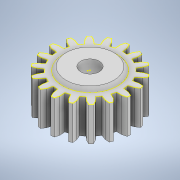
# Autodesk Inventor part: metal_gearbox_gear
Saved by Autodesk Inventor 2020 (Build 240168000, 168)
## iProperties
Created: 2020-01-28
Part Number: metal_gearbox_gear
Material: Generic
Document SubType Name: Modeling
Designer: erwin
Density: 1 g/cm^3
Appearance: Default
Author: erwin
Autodesk Inventor part; units mm, degrees
ref_plane "YZ Plane" through (0, 0, 0) normal (1, 0, 0) x (0, 1, 0)
ref_plane "XZ Plane" through (0, 0, 0) normal (0, 1, 0) x (-1, 0, 0)
ref_plane "XY Plane" through (0, 0, 0) normal (0, 0, 1) x (1, 0, 0)
sketch "Sketch1" plane through (0, 0, 0) normal (0, 1, 0) x (-1, 0, 0)
  line L0 (-38.3271, 50.3843) -> (32.9901, 50.3843) construction
  line L1 (32.9901, 50.3843) -> (32.9901, -44.7054) construction
  line L2 (32.9901, -44.7054) -> (-38.3271, -44.7054) construction
  line L3 (-38.3271, -44.7054) -> (-38.3271, 50.3843) construction
  circle A0 centre (-0.1536, -0.2457) radius 1.55
  arc A1 (6.806, -0.9968) -> (6.8429, -0.4678) centre (-0.1536, -0.2457) ccw
  circle A2 centre (-0.1536, -0.2457) radius 3.9907
  circle A3 centre (-0.1536, -0.2457) radius 4.6909
  circle A4 centre (-0.1536, -0.2457) radius 5.4294
  line L4 (5.1931, -1.1899) -> (6.0958, -1.1899)
  line L5 (6.0958, -1.1899) -> (6.806, -0.9968)
  line L6 (6.8429, -0.4678) -> (6.1696, -0.1708)
  line L7 (5.2729, -0.0666) -> (6.1696, -0.1708)
  line L8 (5.1936, 0.6958) -> (6.0419, 1.0045)
  line L9 (4.8844, 1.7785) -> (5.7626, 1.9874)
  line L10 (6.4969, 1.9385) -> (5.7626, 1.9874)
  arc A5 (6.6432, 1.4288) -> (6.4969, 1.9385) centre (-0.1536, -0.2457) ccw
  line L11 (6.0419, 1.0045) -> (6.6432, 1.4288)
  line L12 (4.5491, 2.4678) -> (5.2407, 3.0481)
  line L13 (3.8882, 3.3796) -> (4.6421, 3.8762)
  line L14 (5.3488, 4.0814) -> (4.6421, 3.8762)
  arc A6 (5.6606, 3.6524) -> (5.3488, 4.0814) centre (-0.1536, -0.2457) ccw
  line L15 (5.2407, 3.0481) -> (5.6606, 3.6524)
  line L16 (3.3375, 3.9126) -> (3.7888, 4.6944)
  line L17 (2.4046, 4.5433) -> (2.9431, 5.2678)
  line L18 (3.537, 5.7024) -> (2.9431, 5.2678)
  arc A7 (3.9767, 5.4059) -> (3.537, 5.7024) centre (-0.1536, -0.2457) ccw
  line L19 (3.7888, 4.6944) -> (3.9767, 5.4059)
  line L20 (1.7047, 4.8559) -> (1.8615, 5.7449)
  line L21 (0.6124, 5.1295) -> (0.8707, 5.9945)
  line L22 (1.2801, 6.6059) -> (0.8707, 5.9945)
  arc A8 (1.7947, 6.4777) -> (1.2801, 6.6059) centre (-0.1536, -0.2457) ccw
  line L23 (1.8615, 5.7449) -> (1.7947, 6.4777)
  line L24 (-0.1522, 5.1838) -> (-0.3089, 6.0728)
  line L25 (-1.2722, 5.0673) -> (-1.3254, 5.9685)
  line L26 (-1.1497, 6.6831) -> (-1.3254, 5.9685)
  arc A9 (-0.6223, 6.7386) -> (-1.1497, 6.6831) centre (-0.1536, -0.2457) ccw
  line L27 (-0.3089, 6.0728) -> (-0.6223, 6.7386)
  line L28 (-2.0093, 4.8568) -> (-2.4606, 5.6386)
  line L29 (-3.0219, 4.3643) -> (-3.3801, 5.193)
  line L30 (-3.4594, 5.9246) -> (-3.3801, 5.193)
  arc A10 (-2.9828, 6.1571) -> (-3.4594, 5.9246) centre (-0.1536, -0.2457) ccw
  line L31 (-2.4606, 5.6386) -> (-2.9828, 6.1571)
  line L32 (-3.6425, 3.9145) -> (-4.334, 4.4947)
  line L33 (-4.4256, 3.1053) -> (-5.0456, 3.7615)
  line L34 (-5.3704, 4.4218) -> (-5.0456, 3.7615)
  arc A11 (-5.0021, 4.8033) -> (-5.3704, 4.4218) centre (-0.1536, -0.2457) ccw
  line L35 (-4.334, 4.4947) -> (-5.0021, 4.8033)
  line L36 (-4.8549, 2.4703) -> (-5.7032, 2.7791)
  line L37 (-5.3141, 1.4421) -> (-6.1211, 1.8466)
  line L38 (-6.6522, 2.3561) -> (-6.1211, 1.8466)
  arc A12 (-6.4366, 2.8406) -> (-6.6522, 2.3561) centre (-0.1536, -0.2457) ccw
  line L39 (-5.7032, 2.7791) -> (-6.4366, 2.8406)
  line L40 (-5.5003, 0.6986) -> (-6.4031, 0.6986)
  line L41 (-5.5801, -0.4247) -> (-6.4768, -0.3205)
  line L42 (-7.1501, -0.0235) -> (-6.4768, -0.3205)
  arc A13 (-7.1132, 0.5055) -> (-7.1501, -0.0235) centre (-0.1536, -0.2457) ccw
  line L43 (-6.4031, 0.6986) -> (-7.1132, 0.5055)
  line L44 (-5.5008, -1.1871) -> (-6.3491, -1.4958)
  line L45 (-5.1916, -2.2699) -> (-6.0699, -2.4787)
  line L46 (-6.8041, -2.4298) -> (-6.0699, -2.4787)
  arc A14 (-6.9504, -1.9201) -> (-6.8041, -2.4298) centre (-0.1536, -0.2457) ccw
  line L47 (-6.3491, -1.4958) -> (-6.9504, -1.9201)
  line L48 (-4.8564, -2.9591) -> (-5.5479, -3.5394)
  line L49 (-4.1955, -3.8709) -> (-4.9493, -4.3675)
  line L50 (-5.656, -4.5727) -> (-4.9493, -4.3675)
  arc A15 (-5.9678, -4.1437) -> (-5.656, -4.5727) centre (-0.1536, -0.2457) ccw
  line L51 (-5.5479, -3.5394) -> (-5.9678, -4.1437)
  line L52 (-3.6447, -4.4039) -> (-4.0961, -5.1857)
  line L53 (-2.7118, -5.0346) -> (-3.2504, -5.7591)
  line L54 (-3.8443, -6.1937) -> (-3.2504, -5.7591)
  arc A16 (-4.284, -5.8972) -> (-3.8443, -6.1937) centre (-0.1536, -0.2457) ccw
  line L55 (-4.0961, -5.1857) -> (-4.284, -5.8972)
  line L56 (-2.0119, -5.3472) -> (-2.1687, -6.2362)
  line L57 (-0.9196, -5.6208) -> (-1.1779, -6.4858)
  line L58 (-1.5873, -7.0973) -> (-1.1779, -6.4858)
  arc A17 (-2.1019, -6.9691) -> (-1.5873, -7.0973) centre (-0.1536, -0.2457) ccw
  line L59 (-2.1687, -6.2362) -> (-2.1019, -6.9691)
  line L60 (-0.155, -5.6751) -> (0.0017, -6.5641)
  line L61 (0.965, -5.5586) -> (1.0181, -6.4598)
  line L62 (0.8425, -7.1744) -> (1.0181, -6.4598)
  arc A18 (0.3151, -7.2299) -> (0.8425, -7.1744) centre (-0.1536, -0.2457) ccw
  line L63 (0.0017, -6.5641) -> (0.3151, -7.2299)
  line L64 (1.702, -5.3482) -> (2.1534, -6.1299)
  line L65 (2.7147, -4.8556) -> (3.0728, -5.6843)
  line L66 (3.1522, -6.4159) -> (3.0728, -5.6843)
  arc A19 (2.6756, -6.6484) -> (3.1522, -6.4159) centre (-0.1536, -0.2457) ccw
  line L67 (2.1534, -6.1299) -> (2.6756, -6.6484)
  line L68 (3.3353, -4.4058) -> (4.0268, -4.986)
  line L69 (4.1184, -3.5966) -> (4.7384, -4.2528)
  line L70 (5.0632, -4.9131) -> (4.7384, -4.2528)
  arc A20 (4.6949, -5.2946) -> (5.0632, -4.9131) centre (-0.1536, -0.2457) ccw
  line L71 (4.0268, -4.986) -> (4.6949, -5.2946)
  line L72 (4.5477, -2.9616) -> (5.396, -3.2704)
  line L73 (5.0069, -1.9334) -> (5.8139, -2.3379)
  line L74 (6.3449, -2.8474) -> (5.8139, -2.3379)
  arc A21 (6.1293, -3.3319) -> (6.3449, -2.8474) centre (-0.1536, -0.2457) ccw
  line L75 (5.396, -3.2704) -> (6.1293, -3.3319)
  point P0 (0, 0)
  dimension "d10" = 360
  dimension "d30" = 3.1
  dimension "d33" = 7
  constraints: 144 end point, 36 point on circle, 23 coincident, 21 centre point, 2 equal length, 1 horizontal, 239 other
  measures "d30" diameter of A0
  measures "d33" radius of A1
extrude "Extrusion1" add sketch "Sketch1" along normal blind 2.85 contours L5 L4 A4 L7 L6 A1 | A4 | L73 L74 A21 L75 L72 A4 | A4 L9 L10 A5 L11 L8 | L69 L70 A20 L71 L68 A4 | A4 L13 L14 A6 L15 L12 | L65 L66 A19 L67 L64 A4 | A4 L17 L18 A7 L19 L16 | L61 L62 A18 L63 L60 A4 | A4 L21 L22 A8 L23 L20 | L57 L58 A17 L59 L56 A4 | A4 L25 L26 A9 L27 L24 | L53 L54 A16 L55 L52 A4 | A4 L29 L30 A10 L31 L28 | L49 L50 A15 L51 L48 A4 | A4 L33 L34 A11 L35 L32 | L45 L46 A14 L47 L44 A4 | A4 L37 L38 A12 L39 L36 | L41 L42 A13 L43 L40 A4 | A2 | A3
extrude "Extrusion2" add sketch "Sketch1" along normal blind 3.4 contours A2
draft "FaceDraft1" angle 45 pull direction (0, 1, 0) faces at (-3.7854, 3.0333, 0.3945) fixed edges at (4.1443, 3.4, -0.2457)
mirror "Mirror1" about plane through (0, 0, 0) normal (0, 1, 0) of "Extrusion1", "Extrusion2", "FaceDraft1"
sketch "Sketch2" plane through (0, 2.85, 0) normal (0, 1, 0) x (1, 0, 0)
  circle A0 centre (0.1536, 0.2457) radius 4.5407 projected
  arc A1 (4.4256, -3.1053) -> (4.8549, -2.4703) centre (0.1536, 0.2457) ccw projected
  line L0 (4.8549, -2.4703) -> (5.7032, -2.7791) projected
  line L1 (5.7032, -2.7791) -> (6.4366, -2.8406) projected
  arc A2 (6.4366, -2.8406) -> (6.6522, -2.3561) centre (0.1536, 0.2457) ccw projected
  line L2 (6.6522, -2.3561) -> (6.1211, -1.8466) projected
  line L3 (6.1211, -1.8466) -> (5.3141, -1.4421) projected
  arc A3 (5.3141, -1.4421) -> (5.5003, -0.6986) centre (0.1536, 0.2457) ccw projected
  line L4 (5.5003, -0.6986) -> (6.4031, -0.6986) projected
  line L5 (6.4031, -0.6986) -> (7.1132, -0.5055) projected
  arc A4 (7.1132, -0.5055) -> (7.1501, 0.0235) centre (0.1536, 0.2457) ccw projected
  line L6 (7.1501, 0.0235) -> (6.4768, 0.3205) projected
  line L7 (6.4768, 0.3205) -> (5.5801, 0.4247) projected
  arc A5 (5.5801, 0.4247) -> (5.5008, 1.1871) centre (0.1536, 0.2457) ccw projected
  line L8 (5.5008, 1.1871) -> (6.3491, 1.4958) projected
  line L9 (6.3491, 1.4958) -> (6.9504, 1.9201) projected
  arc A6 (6.9504, 1.9201) -> (6.8041, 2.4298) centre (0.1536, 0.2457) ccw projected
  line L10 (6.8041, 2.4298) -> (6.0699, 2.4787) projected
  line L11 (6.0699, 2.4787) -> (5.1916, 2.2699) projected
  arc A7 (5.1916, 2.2699) -> (4.8564, 2.9591) centre (0.1536, 0.2457) ccw projected
  line L12 (4.8564, 2.9591) -> (5.5479, 3.5394) projected
  line L13 (5.5479, 3.5394) -> (5.9678, 4.1437) projected
  arc A8 (5.9678, 4.1437) -> (5.656, 4.5727) centre (0.1536, 0.2457) ccw projected
  line L14 (5.656, 4.5727) -> (4.9493, 4.3675) projected
  line L15 (4.9493, 4.3675) -> (4.1955, 3.8709) projected
  arc A9 (4.1955, 3.8709) -> (3.6447, 4.4039) centre (0.1536, 0.2457) ccw projected
  line L16 (3.6447, 4.4039) -> (4.0961, 5.1857) projected
  line L17 (4.0961, 5.1857) -> (4.284, 5.8972) projected
  arc A10 (4.284, 5.8972) -> (3.8443, 6.1937) centre (0.1536, 0.2457) ccw projected
  line L18 (3.8443, 6.1937) -> (3.2504, 5.7591) projected
  line L19 (3.2504, 5.7591) -> (2.7118, 5.0346) projected
  arc A11 (2.7118, 5.0346) -> (2.0119, 5.3472) centre (0.1536, 0.2457) ccw projected
  line L20 (2.0119, 5.3472) -> (2.1687, 6.2362) projected
  line L21 (2.1687, 6.2362) -> (2.1019, 6.9691) projected
  arc A12 (2.1019, 6.9691) -> (1.5873, 7.0973) centre (0.1536, 0.2457) ccw projected
  line L22 (1.5873, 7.0973) -> (1.1779, 6.4858) projected
  line L23 (1.1779, 6.4858) -> (0.9196, 5.6208) projected
  arc A13 (0.9196, 5.6208) -> (0.155, 5.6751) centre (0.1536, 0.2457) ccw projected
  line L24 (0.155, 5.6751) -> (-0.0017, 6.5641) projected
  line L25 (-0.0017, 6.5641) -> (-0.3151, 7.2299) projected
  arc A14 (-0.3151, 7.2299) -> (-0.8425, 7.1744) centre (0.1536, 0.2457) ccw projected
  line L26 (-0.8425, 7.1744) -> (-1.0181, 6.4598) projected
  line L27 (-1.0181, 6.4598) -> (-0.965, 5.5586) projected
  arc A15 (-0.965, 5.5586) -> (-1.702, 5.3482) centre (0.1536, 0.2457) ccw projected
  line L28 (-1.702, 5.3482) -> (-2.1534, 6.1299) projected
  line L29 (-2.1534, 6.1299) -> (-2.6756, 6.6484) projected
  arc A16 (-2.6756, 6.6484) -> (-3.1522, 6.4159) centre (0.1536, 0.2457) ccw projected
  line L30 (-3.1522, 6.4159) -> (-3.0728, 5.6843) projected
  line L31 (-3.0728, 5.6843) -> (-2.7147, 4.8556) projected
  arc A17 (-2.7147, 4.8556) -> (-3.3353, 4.4058) centre (0.1536, 0.2457) ccw projected
  line L32 (-3.3353, 4.4058) -> (-4.0268, 4.986) projected
  line L33 (-4.0268, 4.986) -> (-4.6949, 5.2946) projected
  arc A18 (-4.6949, 5.2946) -> (-5.0632, 4.9131) centre (0.1536, 0.2457) ccw projected
  line L34 (-5.0632, 4.9131) -> (-4.7384, 4.2528) projected
  line L35 (-4.7384, 4.2528) -> (-4.1184, 3.5966) projected
  arc A19 (-4.1184, 3.5966) -> (-4.5477, 2.9616) centre (0.1536, 0.2457) ccw projected
  line L36 (-4.5477, 2.9616) -> (-5.396, 3.2704) projected
  line L37 (-5.396, 3.2704) -> (-6.1293, 3.3319) projected
  arc A20 (-6.1293, 3.3319) -> (-6.3449, 2.8474) centre (0.1536, 0.2457) ccw projected
  line L38 (-6.3449, 2.8474) -> (-5.8139, 2.3379) projected
  line L39 (-5.8139, 2.3379) -> (-5.0069, 1.9334) projected
  arc A21 (-5.0069, 1.9334) -> (-5.1931, 1.1899) centre (0.1536, 0.2457) ccw projected
  line L40 (-5.1931, 1.1899) -> (-6.0958, 1.1899) projected
  line L41 (-6.0958, 1.1899) -> (-6.806, 0.9968) projected
  arc A22 (-6.806, 0.9968) -> (-6.8429, 0.4678) centre (0.1536, 0.2457) ccw projected
  line L42 (-6.8429, 0.4678) -> (-6.1696, 0.1708) projected
  line L43 (-6.1696, 0.1708) -> (-5.2729, 0.0666) projected
  arc A23 (-5.2729, 0.0666) -> (-5.1936, -0.6958) centre (0.1536, 0.2457) ccw projected
  line L44 (-5.1936, -0.6958) -> (-6.0419, -1.0045) projected
  line L45 (-6.0419, -1.0045) -> (-6.6432, -1.4288) projected
  arc A24 (-6.6432, -1.4288) -> (-6.4969, -1.9385) centre (0.1536, 0.2457) ccw projected
  line L46 (-6.4969, -1.9385) -> (-5.7626, -1.9874) projected
  line L47 (-5.7626, -1.9874) -> (-4.8844, -1.7785) projected
  arc A25 (-4.8844, -1.7785) -> (-4.5491, -2.4678) centre (0.1536, 0.2457) ccw projected
  line L48 (-4.5491, -2.4678) -> (-5.2407, -3.0481) projected
  line L49 (-5.2407, -3.0481) -> (-5.6606, -3.6524) projected
  arc A26 (-5.6606, -3.6524) -> (-5.3488, -4.0814) centre (0.1536, 0.2457) ccw projected
  line L50 (-5.3488, -4.0814) -> (-4.6421, -3.8762) projected
  line L51 (-4.6421, -3.8762) -> (-3.8882, -3.3796) projected
  arc A27 (-3.8882, -3.3796) -> (-3.3375, -3.9126) centre (0.1536, 0.2457) ccw projected
  line L52 (-3.3375, -3.9126) -> (-3.7888, -4.6944) projected
  line L53 (-3.7888, -4.6944) -> (-3.9767, -5.4059) projected
  arc A28 (-3.9767, -5.4059) -> (-3.537, -5.7024) centre (0.1536, 0.2457) ccw projected
  line L54 (-3.537, -5.7024) -> (-2.9431, -5.2678) projected
  line L55 (-2.9431, -5.2678) -> (-2.4046, -4.5433) projected
  arc A29 (-2.4046, -4.5433) -> (-1.7047, -4.8559) centre (0.1536, 0.2457) ccw projected
  line L56 (-1.7047, -4.8559) -> (-1.8615, -5.7449) projected
  line L57 (-1.8615, -5.7449) -> (-1.7947, -6.4777) projected
  arc A30 (-1.7947, -6.4777) -> (-1.2801, -6.6059) centre (0.1536, 0.2457) ccw projected
  line L58 (-1.2801, -6.6059) -> (-0.8707, -5.9945) projected
  line L59 (-0.8707, -5.9945) -> (-0.6124, -5.1295) projected
  arc A31 (-0.6124, -5.1295) -> (0.1522, -5.1838) centre (0.1536, 0.2457) ccw projected
  line L60 (0.1522, -5.1838) -> (0.3089, -6.0728) projected
  line L61 (0.3089, -6.0728) -> (0.6223, -6.7386) projected
  arc A32 (0.6223, -6.7386) -> (1.1497, -6.6831) centre (0.1536, 0.2457) ccw projected
  line L62 (1.1497, -6.6831) -> (1.3254, -5.9685) projected
  line L63 (1.3254, -5.9685) -> (1.2722, -5.0673) projected
  arc A33 (1.2722, -5.0673) -> (2.0093, -4.8568) centre (0.1536, 0.2457) ccw projected
  line L64 (2.0093, -4.8568) -> (2.4606, -5.6386) projected
  line L65 (2.4606, -5.6386) -> (2.9828, -6.1571) projected
  arc A34 (2.9828, -6.1571) -> (3.4594, -5.9246) centre (0.1536, 0.2457) ccw projected
  line L66 (3.4594, -5.9246) -> (3.3801, -5.193) projected
  line L67 (3.3801, -5.193) -> (3.0219, -4.3643) projected
  arc A35 (3.0219, -4.3643) -> (3.6425, -3.9145) centre (0.1536, 0.2457) ccw projected
  line L68 (3.6425, -3.9145) -> (4.334, -4.4947) projected
  line L69 (4.334, -4.4947) -> (5.0021, -4.8033) projected
  arc A36 (5.0021, -4.8033) -> (5.3704, -4.4218) centre (0.1536, 0.2457) ccw projected
  line L70 (5.3704, -4.4218) -> (5.0456, -3.7615) projected
  line L71 (5.0456, -3.7615) -> (4.4256, -3.1053) projected
  point P0 (0, 0)
body "Solid1"
